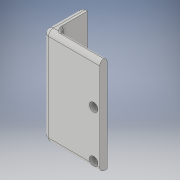
# Autodesk Inventor part: Limit_Switch_Bracket
Saved by Autodesk Inventor 2019.4 (Build 234330000, 330)
## iProperties
Created: 2020-03-06
Part Number: Limit_Switch_Bracket
Material: Generic
Document SubType Name: Modeling
Designer: Jorian Bruslind
Density: 1 g/cm^3
Appearance: Default
Author: Jorian Bruslind
Autodesk Inventor part; units mm, degrees
ref_plane "YZ Plane" through (0, 0, 0) normal (1, 0, 0) x (0, 1, 0)
ref_plane "XZ Plane" through (0, 0, 0) normal (0, 1, 0) x (-1, 0, 0)
ref_plane "XY Plane" through (0, 0, 0) normal (0, 0, 1) x (1, 0, 0)
sketch "Sketch1" plane through (0, 0, 0) normal (0, 1, 0) x (-1, 0, 0)
  line L0 (-10, 1.5) -> (10, 1.5)
  line L1 (10, 1.5) -> (10, -1.5)
  line L2 (10, -1.5) -> (-10, -1.5)
  line L3 (-10, -1.5) -> (-10, 1.5)
  line L4 (-10, 1.5) -> (10, -1.5) construction
  line L5 (10, 1.5) -> (-10, -1.5) construction
  line L6 (10, 1.5) -> (10, -13.5)
  line L7 (10, -13.5) -> (13, -13.5)
  line L8 (13, -13.5) -> (13, 1.5)
  line L9 (13, 1.5) -> (10, 1.5)
  point P0 (0, 0)
  dimension "d0" = 20
  dimension "d1" = 3
  dimension "d2" = 15
  dimension "d3" = 3
  constraints: 20 end point, 4 parallel, 2 midpoint, 2 perpendicular, 1 horizontal, 1 point on line
  measures "d0" distance of L0.start L0.end
  measures "d1" distance of L0.end L1.end
  measures "d2" distance of L0.end L6.end
  measures "d3" distance of L7.end L6.end
extrude "Extrusion1" add sketch "Sketch1" along normal blind 40
sketch "Sketch2" plane through (10, 0, -1.5) normal (0, 0, -1) x (-1, 0, 0)
  line L0 (0, 0) -> (23, 0) projected
  line L1 (0, 0) -> (2.5, 0)
  line L2 (2.5, 0) -> (2.5, 3)
  line L3 (2.5, 0) -> (5.5, 0) construction
  circle A0 centre (2.5, 3) radius 1.75
  line L4 (2.5, 3) -> (2.5, 22.175)
  line L5 (2.5, 3) -> (21.675, 3) construction
  circle A1 centre (2.5, 22.175) radius 1.75
  point P0 (10, 0)
  dimension "d6" = 2.5
  dimension "d7" = 3
  dimension "d8" = 90
  dimension "d9" = 3.5
  dimension "d10" = 19.175
  dimension "d11" = 90
  dimension "d12" = 3.5
  constraints: 10 end point, 2 centre point, 2 coincident, 2 horizontal, 2 perpendicular, 2 vertical, 1 point on line
  measures "d6" distance of L0.start L1.end
  measures "d7" distance of L1.end L2.end
  measures "d8" angle of L3 L2
  measures "d9" diameter of A0
  measures "d10" distance of L4.start L4.end
  measures "d11" angle of L5 L4
  measures "d12" diameter of A1
extrude "Extrusion2" cut sketch "Sketch2" against normal blind 3
fillet "Fillet1" radius 2 3 edges at (-13, 20, -13.5) (-13, 0, -6) (-13, 40, -6)
fillet "Fillet2" radius 2 6 edges at (0, 40, -1.5) (-12.4142, 39.4142, 1.5) (-13, 20, 1.5) (-12.4142, 0.5858, 1.5) (-0.5, 0, 1.5) (-0.5, 40, 1.5)
fillet "Fillet3" radius 2 2 edges at (-10, 39.2247, -1.0811) (-10, 19, -1.5)
sketch "Sketch3" plane through (-13, 2, -11.5) normal (-1, 0, 0) x (0, 0, 1)
  line L0 (-2, -2) -> (-2, 38) projected
  line L1 (-2, -2) -> (-2, 18)
  line L2 (-2, 18) -> (4.5, 18)
  line L3 (-2, -2) -> (11, -2) projected
  line L4 (4.5, 18) -> (4.5, 13)
  line L5 (4.5, 18) -> (9.5, 18) construction
  line L6 (4.5, 18) -> (4.5, 23)
  line L7 (4.5, 18) -> (9.5, 18) construction
  circle A0 centre (4.5, 13) radius 1.75
  circle A1 centre (4.5, 23) radius 1.75
  point P0 (11.5, -2)
  dimension "d18" = 5
  dimension "d19" = 90
  dimension "d20" = 6.5
  dimension "d21" = 5
  dimension "d22" = 90
  dimension "d23" = 3.5
  dimension "d24" = 3.5
  constraints: 12 end point, 2 centre point, 2 coincident, 2 horizontal, 2 perpendicular, 2 vertical, 1 midpoint, 1 parallel
  measures "d18" distance of L2.end L4.end
  measures "d19" angle of L4 L5
  measures "d20" distance between parallel lines of L0 L4
  measures "d21" distance of L2.end L6.end
  measures "d22" angle of L7 L6
  measures "d23" diameter of A0
  measures "d24" diameter of A1
extrude "Extrusion3" cut sketch "Sketch3" against normal blind 3
body "Solid1"
